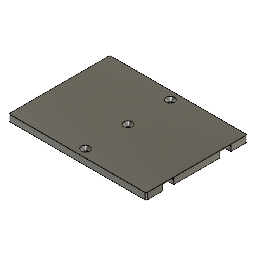
new_mount v2 v2 (Autodesk Fusion 360 design; units mm, degrees)
Autodesk Fusion 360 part; units mm, degrees
sketch "Sketch2" plane through (0, 0, 0) normal (0, 0, -1) x (1, 0, 0)
  arc A0 (124, -92) -> (125, -91) centre (124, -91) ccw
  line L0 (125, -91) -> (125, -1)
  arc A1 (125, -1) -> (124, 0) centre (124, -1) ccw
  line L1 (124, 0) -> (1, 0)
  arc A2 (1, 0) -> (0, -1) centre (1, -1) ccw
  line L2 (0, -1) -> (0, -91)
  arc A3 (0, -91) -> (1, -92) centre (1, -91) ccw
  line L3 (1, -92) -> (124, -92)
  circle A4 centre (54.1, -72.1) radius 1
  circle A5 centre (11, -21.3) radius 1
  circle A6 centre (26.2, -72.1) radius 1
  circle A7 centre (59.2, -20) radius 1
extrude "Extrude1" add sketch "Sketch2" along normal blind 6
sketch "Sketch1" plane through (0, 0, -6) normal (0, 0, -1) x (1, 0, 0)
  circle A0 centre (59.2, -20) radius 1
  circle A1 centre (11, -21.3) radius 1
  circle A2 centre (26.2, -72.1) radius 1
  circle A3 centre (54.1, -72.1) radius 1
  line L0 (1, -92) -> (124, -92)
  arc A4 (124, -92) -> (125, -91) centre (124, -91) ccw
  line L1 (125, -91) -> (125, -1)
  arc A5 (125, -1) -> (124, 0) centre (124, -1) ccw
  line L2 (124, 0) -> (1, 0)
  arc A6 (1, 0) -> (0, -1) centre (1, -1) ccw
  line L3 (0, -1) -> (0, -91)
  arc A7 (0, -91) -> (1, -92) centre (1, -91) ccw
  line L4 (0, -15) -> (125, -15)
  line L5 (125, -15) -> (125, -25)
  line L6 (125, -25) -> (0, -25)
  line L7 (0, -25) -> (0, -15)
  line L8 (0, -67) -> (125, -67)
  line L9 (125, -67) -> (125, -77)
  line L10 (125, -77) -> (0, -77)
  line L11 (0, -77) -> (0, -67)
  dimension "d215" = 15
  dimension "d216" = 10
  dimension "d217" = 15
  dimension "d218" = 10
  constraint horizontal L4
  constraint vertical L5
  constraint horizontal L6
  constraint vertical L7
  constraint coincident L1 L5.end
  constraint coincident L3 L4.start
  constraint horizontal L8
  constraint vertical L9
  constraint horizontal L10
  constraint vertical L11
  constraint coincident L1 L9.end
  constraint coincident L3 L8.start
  measures "d215" distance of L2 L4
  measures "d216" distance of L4.start L6.end
  measures "d217" distance of L0 L10
  measures "d218" distance of L8.start L10.end
extrude "Extrude2" cut sketch "Sketch1" against normal blind 3 contours L1 L3 L8 L9 L10 L11 | L1 L3 L4 L5 L6 L7
fillet "Fillet1" radius 3 1 edges at (125, 20, -3)
fillet "Fillet2" radius 3 1 edges at (125, 72, -3)
fillet "Fillet3" radius 3 1 edges at (0, 72, -3)
fillet "Fillet4" radius 3 1 edges at (0, 20, -3)
delete_face "DeleteFace1" 1 faces at (60.1215, 19.6116, -2)
delete_face "DeleteFace2" 1 faces at (11.995, 21.3996, -1)
delete_face "DeleteFace3" 1 faces at (25.2198, 71.9019, -2)
delete_face "DeleteFace4" 1 faces at (55.0691, 71.8532, -2)
hole "Hole1" at (62.5, 46, 0) direction (0, 0, -1) diameter 2.5 end through all countersink diameter 7.5 countersink angle 90
hole "Hole2" at (62.5, 7.5, 0) direction (0, 0, -1) diameter 2.5 end through all countersink diameter 7.5 countersink angle 90
hole "Hole3" at (62.5, 84.5, 0) direction (0, 0, -1) diameter 2.5 end through all countersink diameter 7.5 countersink angle 90
